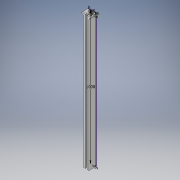
# Autodesk Inventor part: Fuehrungsschiene
Saved by Autodesk Inventor 2017 (Build 210142000, 142)
## iProperties
Part Number: Fuehrungsschiene
Material: Generisch
Document SubType Name: Modeling
Designer: Julian
Density: 1 g/cm^3
Appearance: Vorgabe
Author: Julian
Autodesk Inventor part; units mm, degrees
ref_plane "YZ Plane" through (0, 0, 0) normal (1, 0, 0) x (0, 1, 0)
ref_plane "XZ Plane" through (0, 0, 0) normal (0, 1, 0) x (-1, 0, 0)
ref_plane "XY Plane" through (0, 0, 0) normal (0, 0, 1) x (1, 0, 0)
sketch "Skizze1" plane through (0, 0, 0) normal (0, 1, 0) x (-1, 0, 0)
  line L0 (0, 0) -> (30, 0)
  line L1 (30, 0) -> (30, -1000)
  line L2 (30, -1000) -> (0, -1000)
  line L3 (0, -1000) -> (0, 0)
  line L4 (0, 0) -> (-20, 0)
  line L5 (-5, -20) -> (0, -20)
  arc A0 (0, -20) -> (-20, 0) centre (-20, -20) ccw
  line L6 (30, 0) -> (30, -20)
  line L7 (30, -20) -> (35, -20)
  arc A1 (50, 0) -> (30, -20) centre (50, -20) ccw
  line L8 (50, 0) -> (50, -5)
  arc A2 (50, -5) -> (35, -20) centre (50, -20) ccw
  line L9 (0, -20) -> (-5, -20)
  arc A3 (-5, -20) -> (-20, -5) centre (-20, -20) ccw
  line L10 (35, -20) -> (35, -1000)
  line L11 (35, -1000) -> (30, -1000)
  line L12 (0, -1000) -> (-5, -1000)
  line L13 (-5, -1000) -> (-5, -20)
  line L14 (30, 0) -> (50, 0)
  line L15 (-20, -5) -> (-20, 0)
  line L16 (-20, 0) -> (0, 0)
  line L17 (0, 0) -> (0, -20)
  line L18 (0, -20) -> (-5, -20)
  line L19 (-20, -5) -> (-20, 0)
  arc A4 (0, -20) -> (-20, 0) centre (-20, -20) ccw
  line L20 (0, -20) -> (0, 0)
  line L21 (0, 0) -> (-20, 0)
  dimension "d0" = 30
  dimension "d1" = 1000
  dimension "d2" = 20
  dimension "d5" = 20
  dimension "d10" = 5
  dimension "d11" = 5
  dimension "d12" = 5
  constraints: 44 end point, 10 point on circle, 9 perpendicular, 5 centre point, 5 collinear, 5 point on line, 3 coincident, 3 horizontal, 2 tangent, 2 vertical
  measures "d0" distance of L0.start L0.end
  measures "d1" distance of L0.end L1.end
  measures "d2" distance of L0.start L4.end
  measures "d5" distance of L0.end L6.end
  measures "d10" distance of L8.start L8.end
  measures "d11" distance of L5.start L9.start
  measures "d12" distance of L2.end L12.end
extrude "Extrusion1" add sketch "Skizze1" along normal blind 5
extrude "Extrusion2" add sketch "Skizze1" against normal blind 50 contours L3 L12 L13 L5 | L5 A3 L15 A0 | L7 L10 L11 L1 | A1 L8 A2 L7
extrude "Extrusion3" add sketch "Skizze1" against normal blind 50 contours L0 L1 L2 L3 | L3 A0 L4 | L14 A1 L1
extrude "Extrusion4" cut sketch "Skizze1" against normal blind 40 contours L0 L1 L2 L3 | L3 A0 L4 | L14 A1 L1
sketch "Skizze2" plane through (0, 0, 0) normal (0, -1, 0) x (1, 0, 0)
  arc A0 (-35, -20) -> (-50, -5) centre (-50, -20) ccw projected
  line L0 (5, -20) -> (5, -1000) projected
  line L1 (-50, -5) -> (5, -20)
  line L2 (5, -36.012) -> (-15, -36.012)
  line L3 (-35, -20) -> (-35, -1000) projected
  line L4 (-15, -36.012) -> (-22.5, -36.012)
  line L5 (-22.5, -36.012) -> (-7.5, -36.012)
  line L6 (-7.5, -36.012) -> (-7.5, 0)
  line L7 (-50, 0) -> (20, 0) projected
  line L8 (-7.5, 0) -> (-22.5, 0)
  line L9 (-22.5, 0) -> (-22.5, -1000)
  line L10 (-30, -1000) -> (0, -1000) projected
  line L11 (-22.5, -1000) -> (-7.5, -1000)
  line L12 (-7.5, -1000) -> (-7.5, 0)
  point P0 (0, 0)
  dimension "d21" = 20
  dimension "d22" = 15
  dimension "d23" = 15
  dimension "d24" = 15
  constraints: 18 end point, 7 point on line, 3 perpendicular
  measures "d21" distance of L2.start L2.end
  measures "d22" distance of L4.end L5.end
  measures "d23" distance of L6.end L8.end
  measures "d24" distance of L9.end L11.end
extrude "Extrusion5" cut sketch "Skizze2" along normal blind 50 contours L9 L7 L6 L1 | L1 L6 L2 L4 L9 | L4 L2 L12 L10 L9
